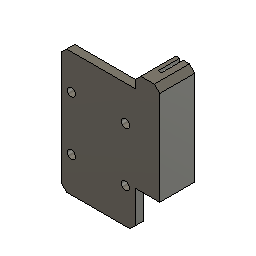
Placestation_Toolhead (Autodesk Fusion 360 archive; units mm, degrees)
design "Z-gantry-backplate-left-mgn12h"
part number: MGN12H-linear-rail-carriage
Autodesk Fusion 360 part; units mm, degrees
note: some values were not read from the file. Set by a fixed rule: which face or edge a step refers to.
sketch "Sketch4" plane through (0, 0, 122.6176) normal (0, 0, 1) x (1, 0, 0)
  line L0 (15.9, 225.325) -> (3.9, 225.325)
  line L1 (3.9, 225.325) -> (3.9, 192.925)
  line L2 (3.9, 192.925) -> (15.9, 192.925)
  line L3 (15.9, 192.925) -> (15.9, 225.325)
  line L4 (41.5656, 188.8314, 7.825) -> (5.0656, 188.8314, 7.825)
  line L5 (5.0656, 188.8314, 7.825) -> (5.0656, 234.6853, 9.8822)
  line L6 (5.0656, 234.6853, 9.8822) -> (41.5656, 234.6853, 9.8822)
  line L7 (41.5656, 234.6853, 9.8822) -> (41.5656, 188.8314, 7.825)
  line L8 (41.5656, 188.8314, 7.825) -> (5.0656, 234.6853, 9.8822) construction
  line L9 (5.0656, 188.8314, 7.825) -> (41.5656, 234.6853, 9.8822) construction
  line L10 (23.4, 192.925, -0.2) -> (23.4, 225.325, -0.2)
  circle A0 through (21.45, 219.125, 0.1295) (19.125, 220.4673, 0.1295) (19.125, 217.7827, 0.1295)
  circle A1 through (21.1295, 219.125, 0.1295) (19.2852, 220.1898, 0.1295) (19.2852, 218.0602, 0.1295)
  circle A2 through (1.45, 219.125, 0.1295) (-0.875, 220.4673, 0.1295) (-0.875, 217.7827, 0.1295)
  circle A3 through (1.1295, 219.125, 0.1295) (-0.7147, 220.1898, 0.1295) (-0.7147, 218.0602, 0.1295)
  circle A4 through (21.45, 199.125, 0.1295) (19.125, 200.4673, 0.1295) (19.125, 197.7827, 0.1295)
  circle A5 through (21.1295, 199.125, 0.1295) (19.2852, 200.1898, 0.1295) (19.2852, 198.0602, 0.1295)
  circle A6 through (1.45, 199.125, 0.1295) (-0.875, 200.4673, 0.1295) (-0.875, 197.7827, 0.1295)
  circle A7 through (1.1295, 199.125, 0.1295) (-0.7147, 200.1898, 0.1295) (-0.7147, 198.0602, 0.1295)
  point P0 (23.3156, 211.7584)
  point P1 (23.3156, 211.7584)
  dimension "d15" = 16.2
  dimension "d17" = 36.5
  dimension "d18" = 45.9
  dimension "d19" = 9.054
  dimension "d21" = 3.1
  dimension "d22" = 3.1
  dimension "d23" = 3.1
  dimension "d24" = 3.1
  constraint coincident P1 P0
  measures "d15" distance of L0 P1
sketch "Sketch5" plane through (10.1103, 0, 115.5608) normal (-0.087156, 0, -0.996195) x (-0.996195, 0, 0.087156)
  line L0 (5.3253, 232.125) -> (4.9573, 232.125)
  line L1 (4.9573, 232.125) -> (4.9573, 186.125)
  line L2 (4.9573, 186.125) -> (5.3253, 186.125)
  line L3 (5.3253, 186.125) -> (5.3253, 232.125)
sketch "Sketch6" plane through (0, 0, 123.0176) normal (0, 0, 1) x (1, 0, 0)
  line L0 (22.8, 225.325) -> (16.3, 225.325)
  line L1 (16.3, 225.325) -> (16.3, 192.925)
  line L2 (16.3, 192.925) -> (22.8, 192.925)
  line L3 (22.8, 192.925) -> (22.8, 225.325)
  circle A0 centre (19.9, 219.125) radius 1.5
  circle A1 centre (19.9, 199.125) radius 1.5
sketch "Sketch7" plane through (0, 0, 123.0176) normal (0, 0, 1) x (1, 0, 0)
  line L0 (3.5, 225.325) -> (-3, 225.325)
  line L1 (-3, 225.325) -> (-3, 192.925)
  line L2 (-3, 192.925) -> (3.5, 192.925)
  line L3 (3.5, 192.925) -> (3.5, 225.325)
  circle A0 centre (-0.1, 219.125) radius 1.5
  circle A1 centre (-0.1, 199.125) radius 1.5
sketch "Sketch8" plane through (0, -5.461, 121.726) normal (0, 0.044818, -0.998995) x (-1, 0, 0)
  line L0 (-5.0656, 240.3879) -> (-41.5656, 240.3879)
  line L1 (-41.5656, 240.3879) -> (-41.5656, 194.4879)
  line L2 (-41.5656, 194.4879) -> (-5.0656, 194.4879)
  line L3 (-5.0656, 194.4879) -> (-5.0656, 240.3879)
  line L4 (-41.5656, 235.3879) -> (-33.6656, 235.3879)
  line L5 (-33.6656, 235.3879) -> (-33.6656, 194.4879)
  line L6 (-33.6656, 194.4879) -> (-41.5656, 194.4879)
  line L7 (-41.5656, 194.4879) -> (-41.5656, 235.3879)
  line L8 (-39.5659, 194.4879) -> (-41.5656, 196.4876)
  line L9 (-39.5659, 194.4879) -> (-32.9811, 194.4879) construction
  line L10 (-35.6653, 194.4879) -> (-33.6656, 196.4876)
  line L11 (-35.6653, 194.4879) -> (-22.4855, 194.4879) construction
  line L12 (-39.5659, 240.3879) -> (-41.5656, 238.3882)
  line L13 (-39.5659, 240.3879) -> (-32.2699, 240.3879) construction
  dimension "d33" = 7.9
  dimension "d34" = 40.9
  dimension "d36" = 5
  dimension "d37" = 45
  dimension "d38" = 2.828
  dimension "d39" = 45
  dimension "d40" = 2.828
  dimension "d41" = 45
  dimension "d42" = 2.828
  constraint horizontal L4
  constraint vertical L5
  constraint horizontal L6
  constraint vertical L7
  constraint coincident L1 L4.start
  constraint horizontal L9
  constraint coincident L2 L8.start
  constraint coincident L1 L8.end
  constraint horizontal L11
  constraint coincident L2 L10.start
  constraint coincident L5 L10.end
  constraint horizontal L13
  constraint coincident L0 L12.start
  constraint coincident L1 L12.end
  measures "d33" distance of L4.start L4.end
  measures "d34" distance of L4.start L1.end
  measures "d36" distance of L0 L4
  measures "d37" angle of L8 L9
  measures "d38" distance of L8.start L8.end
  measures "d39" angle of L10 L11
  measures "d40" distance of L10.start L10.end
  measures "d41" angle of L12 L13
  measures "d42" distance of L12.start L12.end
sketch "Sketch9" plane through (0, 235.1513, 10.5496) normal (0, 0.998995, 0.044818) x (-1, 0, 0)
  line L0 (-41.5656, 121.8485) -> (-41.5656, 111.8485)
  line L1 (-41.5656, 111.8485) -> (-33.6656, 111.8485)
  line L2 (-33.6656, 111.8485) -> (-33.6656, 121.8485)
  circle A0 centre (-27.5974, 117.8274) radius 1.575
  circle A1 centre (-27.5974, 117.8274) radius 1.25
  line L3 (-33.6656, 121.8485) -> (-41.5656, 121.8485)
  dimension "d52" = 3.15
  dimension "d53" = 2.5
  constraint concentric A0 A1
  measures "d52" diameter of A0
  measures "d53" diameter of A1
sketch "Sketch10" plane through (0, -5.461, 121.726) normal (0, 0.044818, -0.998995) x (-1, 0, 0)
  line L0 (-39.5659, 240.3879) -> (-41.5656, 238.3882)
  line L1 (-41.5656, 238.3882) -> (-41.5656, 235.3879)
  line L2 (-41.5656, 235.3879) -> (-33.6656, 235.3879)
  line L3 (-33.6656, 235.3879) -> (-33.6656, 196.4876)
  line L4 (-33.6656, 196.4876) -> (-35.6653, 194.4879)
  line L5 (-35.6653, 194.4879) -> (-5.0656, 194.4879)
  line L6 (-5.0656, 194.4879) -> (-5.0656, 240.3879)
  line L7 (-5.0656, 240.3879) -> (-39.5659, 240.3879)
  line L8 (-7.0653, 194.4879) -> (-5.0656, 196.4876)
  line L9 (-7.0653, 194.4879) -> (-6.662, 194.4879) construction
  dimension "d57" = 45
  dimension "d58" = 2.828
  constraint horizontal L9
  constraint coincident L5 L8.start
  constraint coincident L6 L8.end
  measures "d57" angle of L8 L9
  measures "d58" distance of L8.start L8.end
sketch "Sketch11" plane through (0, -5.461, 121.726) normal (0, 0.044818, -0.998995) x (-1, 0, 0)
  line L0 (-39.5659, 240.3879) -> (-41.5656, 238.3882)
  line L1 (-41.5656, 238.3882) -> (-41.5656, 235.3879)
  line L2 (-41.5656, 235.3879) -> (-33.6656, 235.3879)
  line L3 (-33.6656, 235.3879) -> (-33.6656, 196.4876)
  line L4 (-33.6656, 196.4876) -> (-35.6653, 194.4879)
  line L5 (-35.6653, 194.4879) -> (-5.0656, 194.4879)
  line L6 (-5.0656, 194.4879) -> (-5.0656, 240.3879)
  line L7 (-5.0656, 240.3879) -> (-39.5659, 240.3879)
  line L8 (-5.0656, 204.4879) -> (-14.0656, 204.4879)
  line L9 (-14.0656, 204.4879) -> (-14.0656, 245.3879)
  line L10 (-14.0656, 245.3879) -> (-5.0656, 245.3879)
  line L11 (-5.0656, 245.3879) -> (-5.0656, 204.4879)
  line L12 (-7.0653, 204.4879) -> (-5.0656, 206.4876)
  line L13 (-7.0653, 204.4879) -> (12.9274, 204.4879) construction
  line L14 (-14.0656, 243.3882) -> (-12.0659, 245.3879)
  line L15 (-14.0656, 243.3882) -> (6.6806, 243.3882) construction
  line L16 (-5.0656, 243.3882) -> (-7.0653, 245.3879)
  line L17 (-5.0656, 243.3882) -> (10.0246, 243.3882) construction
  line L18 (-16.0653, 240.3879) -> (-14.0656, 242.3876)
  line L19 (-16.0653, 240.3879) -> (5.0782, 240.3879) construction
  dimension "d64" = 9
  dimension "d65" = 40.9
  dimension "d66" = 10
  dimension "d67" = 45
  dimension "d68" = 2.828
  dimension "d69" = 45
  dimension "d70" = 2.828
  dimension "d71" = 45
  dimension "d72" = 2.828
  dimension "d75" = 45
  dimension "d76" = 2.828
  constraint horizontal L8
  constraint vertical L9
  constraint horizontal L10
  constraint vertical L11
  constraint coincident L6 L8.start
  constraint horizontal L13
  constraint coincident L8 L12.start
  constraint coincident L6 L12.end
  constraint horizontal L15
  constraint coincident L9 L14.start
  constraint coincident L10 L14.end
  constraint horizontal L17
  constraint coincident L11 L16.start
  constraint coincident L10 L16.end
  constraint horizontal L19
  constraint coincident L7 L18.start
  constraint coincident L9 L18.end
  measures "d64" distance of L8.start L8.end
  measures "d65" distance of L8.start L10.end
  measures "d66" distance of L5 L8
  measures "d67" angle of L12 L13
  measures "d68" distance of L12.start L12.end
  measures "d69" angle of L14 L15
  measures "d70" distance of L14.start L14.end
  measures "d71" angle of L16 L17
  measures "d72" distance of L16.start L16.end
  measures "d75" angle of L18 L19
  measures "d76" distance of L18.start L18.end
sketch "Sketch12" plane through (0, -5.0128, 111.7361) normal (0, 0.044818, -0.998995) x (-1, 0, 0)
  line L0 (-5.0656, 206.4876) -> (-5.0656, 243.3882)
  line L1 (-5.0656, 243.3882) -> (-7.0653, 245.3879)
  line L2 (-7.0653, 245.3879) -> (-12.0659, 245.3879)
  line L3 (-12.0659, 245.3879) -> (-14.0656, 243.3882)
  line L4 (-14.0656, 243.3882) -> (-14.0656, 204.4879)
  line L5 (-14.0656, 204.4879) -> (-7.0653, 204.4879)
  line L6 (-7.0653, 204.4879) -> (-5.0656, 206.4876)
  line L7 (-10.6656, 245.3879) -> (-9.3656, 245.3879)
  line L8 (-9.3656, 245.3879) -> (-9.3656, 204.4879)
  line L9 (-9.3656, 204.4879) -> (-10.6656, 204.4879)
  line L10 (-10.6656, 204.4879) -> (-10.6656, 245.3879)
  dimension "d81" = 1.3
  dimension "d82" = 40.9
  dimension "d83" = 3.4
  constraint horizontal L7
  constraint vertical L8
  constraint horizontal L9
  constraint vertical L10
  constraint coincident L2 L7.start
  measures "d81" distance of L7.start L7.end
  measures "d82" distance of L7.start L9.end
  measures "d83" distance of L4 L10
sketch "Sketch13" plane through (0, -5.0128, 111.7361) normal (0, 0.044818, -0.998995) x (-1, 0, 0)
  line L0 (-9.3656, 245.3879) -> (-9.3656, 204.4879)
  line L1 (-9.3656, 204.4879) -> (-7.0653, 204.4879)
  line L2 (-7.0653, 204.4879) -> (-5.0656, 206.4876)
  line L3 (-5.0656, 206.4876) -> (-5.0656, 243.3882)
  line L4 (-5.0656, 243.3882) -> (-7.0653, 245.3879)
  line L5 (-7.0653, 245.3879) -> (-9.3656, 245.3879)
  arc A0 (-9.3656, 245.3879) -> (-9.3656, 244.3879) centre (-9.3656, 244.8879) ccw
  arc A1 (-9.3656, 245.3879) -> (-9.3656, 244.3879) centre (-9.349, 244.8879) ccw
  dimension "d86" = 1
  dimension "d87" = 1
  constraint tangent L5 A0
  constraint coincident L0.start L5.end
  constraint coincident L0 L5.end
  measures "d86" distance of L0.start A0.end
  measures "d87" distance of A0.end L0.start
pattern_linear "R-Pattern2" [no effect]
sketch "Sketch14" plane through (0, -5.461, 121.726) normal (0, 0.044818, -0.998995) x (-1, 0, 0)
  line L0 (-14.0656, 243.3882) -> (-14.0656, 242.3876)
  line L1 (-14.0656, 242.3876) -> (-16.0653, 240.3879)
  line L2 (-14.0656, 243.3882) -> (-14.0656, 194.4879)
  line L3 (-14.0656, 202.4882) -> (-12.0659, 204.4879)
  line L4 (-14.0656, 202.4882) -> (6.6806, 202.4882) construction
  line L5 (-16.0653, 194.4879) -> (-14.0656, 196.4876)
  line L6 (-16.0653, 194.4879) -> (4.3386, 194.4879) construction
  line L7 (-12.0659, 204.4879) -> (-7.0653, 204.4879)
  line L8 (-7.0653, 204.4879) -> (-5.0656, 206.4876)
  line L9 (-5.0656, 206.4876) -> (-5.0656, 194.4879)
  line L10 (-5.0656, 194.4879) -> (-14.0656, 194.4879)
  line L11 (-16.0653, 240.3879) -> (-5.0656, 240.3879)
  line L12 (-5.0656, 243.3882) -> (-7.0653, 245.3879)
  line L13 (-7.0653, 245.3879) -> (-12.0659, 245.3879)
  line L14 (-12.0659, 245.3879) -> (-14.0656, 243.3882)
  line L15 (-5.0656, 240.3879) -> (-5.0656, 243.3882)
  dimension "d101" = 45
  dimension "d102" = 2.828
  dimension "d103" = 45
  dimension "d104" = 2.828
  constraint coincident L0.start L2.start
  constraint horizontal L4
  constraint coincident L2 L3.start
  constraint horizontal L6
  constraint coincident L2 L5.end
  measures "d101" angle of L3 L4
  measures "d102" distance of L3.start L3.end
  measures "d103" angle of L5 L6
  measures "d104" distance of L5.start L5.end
sketch "1st for left Sketch" plane through (0, 0, 122.6176) normal (0, 0, 1) x (1, 0, 0)
  line L0 (15.9, 225.325) -> (3.9, 225.325)
  line L1 (3.9, 225.325) -> (3.9, 192.925)
  line L2 (3.9, 192.925) -> (15.9, 192.925)
  line L3 (15.9, 192.925) -> (15.9, 225.325)
  line L4 (23.4, 192.925, -0.2) -> (23.4, 225.325, -0.2)
  line L5 (32.5981, 232.075, -0.0049) -> (-3.9019, 232.075, -0.0049)
  line L6 (-3.9019, 232.075, -0.0049) -> (-3.9019, 186.175, -0.0005)
  line L7 (-3.9019, 186.175) -> (32.5981, 186.175)
  line L8 (32.5981, 186.175, -0.0005) -> (32.5981, 232.075, -0.0049)
  line L9 (32.5981, 232.075, -0.0049) -> (-3.9019, 186.175, -0.0005) construction
  line L10 (-3.9019, 232.075, -0.0049) -> (32.5981, 186.175, -0.0005) construction
  point P0 (14.3481, 209.125)
  point P1 (14.3481, 209.125)
  dimension "d109" = 16.2
  dimension "d110" = 9.054
  dimension "d111" = 36.5
  dimension "d112" = 45.9
  constraint coincident P1 P0
  measures "d109" distance of L0 P1
  measures "d111" distance of L7.start L7.end
sketch "1st for left Sketch (curves on the plane with normal 0, 0.0001, 1 at 0.0173 mm)" plane through (0, 0, 122.6349) normal (0, 0.000096, 1) x (-1, 0, 0)
  line L0 (-32.5981, -232.075) -> (3.9019, -232.075)
  line L1 (3.9019, -232.075) -> (3.9019, -186.175)
  line L2 (3.9019, -186.175) -> (-32.5981, -186.175)
  line L3 (-32.5981, -186.175) -> (-32.5981, -232.075)
  line L4 (-32.5981, -232.075) -> (3.9019, -186.175) construction
  line L5 (3.9019, -232.075) -> (-32.5981, -186.175) construction
extrude "Extrude16" add sketch "1st for left Sketch (curves on the plane with normal 0, 0.0001, 1 at 0.0173 mm)" along normal blind 3
sketch "Sketch16" plane through (0, 0, 123.0176) normal (0, 0, 1) x (1, 0, 0)
  line L0 (3.5, 225.325) -> (-3, 225.325)
  line L1 (-3, 225.325) -> (-3, 192.925)
  line L2 (-3, 192.925) -> (3.5, 192.925)
  line L3 (3.5, 192.925) -> (3.5, 225.325)
  circle A0 centre (-0.1, 219.125) radius 1.5
  circle A1 centre (-0.1, 199.125) radius 1.5
sketch "Sketch17" plane through (0, 0, 123.0176) normal (0, 0, 1) x (1, 0, 0)
  line L0 (22.8, 225.325) -> (16.3, 225.325)
  line L1 (16.3, 225.325) -> (16.3, 192.925)
  line L2 (16.3, 192.925) -> (22.8, 192.925)
  line L3 (22.8, 192.925) -> (22.8, 225.325)
  circle A0 centre (19.9, 219.125) radius 1.5
  circle A1 centre (19.9, 199.125) radius 1.5
extrude "Extrude17" cut sketch "Sketch16" sketch "Sketch17" along normal blind 3 contours A0 | A1 of sketch 2 contours A0 | A1
extrude "Extrude18" cut 4 faces at (-0.5131, 218.6943, 123.0176) (-0.5131, 198.6943, 123.0176) (19.4869, 218.6943, 123.0176) (19.4869, 198.6943, 123.0176) along direction (0, 0, -1) blind 1
sketch "Sketch18" plane through (0, 0.0118, 122.6349) normal (0, -0.000096, -1) x (-1, 0, 0)
  ellipse E0 centre (-19.9, 199.1132) end of major axis (-19.9, 197.6132) minor radius 1.5
  ellipse E1 centre (0.1, 219.1132) end of major axis (0.1, 217.6132) minor radius 1.5
  ellipse E2 centre (-19.9, 219.1132) end of major axis (-19.9, 217.6132) minor radius 1.5
  ellipse E3 centre (0.1, 199.1132) end of major axis (0.1, 197.6132) minor radius 1.5
  line L0 (-32.5981, 232.0632) -> (-32.5981, 186.1632)
  line L1 (-32.5981, 186.1632) -> (3.9019, 186.1632)
  line L2 (3.9019, 186.1632) -> (3.9019, 232.0632)
  line L3 (3.9019, 232.0632) -> (-32.5981, 232.0632)
  line L4 (1.9022, 186.1632) -> (3.9019, 188.1629)
  line L5 (1.9022, 186.1632) -> (3.9019, 186.1632) construction
  line L6 (1.9022, 232.0632) -> (3.9019, 230.0635)
  line L7 (1.9022, 232.0632) -> (5.2821, 232.0632) construction
  line L8 (-30.5985, 186.1632) -> (-32.5981, 188.1629)
  line L9 (-30.5985, 186.1632) -> (-32.7199, 186.1632) construction
  dimension "d119" = 45
  dimension "d120" = 2.828
  dimension "d121" = 45
  dimension "d122" = 2.828
  dimension "d123" = 45
  dimension "d124" = 2.828
  constraint horizontal L5
  constraint coincident L1 L4.start
  constraint coincident L2 L4.end
  constraint horizontal L7
  constraint coincident L3 L6.start
  constraint coincident L2 L6.end
  constraint horizontal L9
  constraint coincident L1 L8.start
  constraint coincident L0 L8.end
  measures "d119" angle of L4 L5
  measures "d120" distance of L4.start L4.end
  measures "d121" angle of L6 L7
  measures "d122" distance of L6.start L6.end
  measures "d123" angle of L8 L9
  measures "d124" distance of L8.start L8.end
extrude "Extrude19" cut sketch "Sketch18" against normal blind 3 contours L0 L1 L8 | L2 L3 L6 | L1 L2 L4
sketch "Sketch19" plane through (0, 0.0118, 122.6349) normal (0, -0.000096, -1) x (-1, 0, 0)
  ellipse E0 centre (0.1, 199.1132) end of major axis (0.1, 197.6132) minor radius 1.5
  ellipse E1 centre (-19.9, 219.1132) end of major axis (-19.9, 217.6132) minor radius 1.5
  ellipse E2 centre (0.1, 219.1132) end of major axis (0.1, 217.6132) minor radius 1.5
  ellipse E3 centre (-19.9, 199.1132) end of major axis (-19.9, 197.6132) minor radius 1.5
  line L0 (-32.5981, 188.1629) -> (-30.5985, 186.1632)
  line L1 (-30.5985, 186.1632) -> (1.9022, 186.1632)
  line L2 (1.9022, 186.1632) -> (3.9019, 188.1629)
  line L3 (3.9019, 188.1629) -> (3.9019, 230.0635)
  line L4 (3.9019, 230.0635) -> (1.9022, 232.0632)
  line L5 (1.9022, 232.0632) -> (-32.5981, 232.0632)
  line L6 (-32.5981, 232.0632) -> (-32.5981, 188.1629)
  line L7 (-32.5981, 237.0632) -> (-23.5981, 237.0632)
  line L8 (-23.5981, 237.0632) -> (-23.5981, 196.1632)
  line L9 (-23.5981, 196.1632) -> (-32.5981, 196.1632)
  line L10 (-32.5981, 196.1632) -> (-32.5981, 237.0632)
  line L11 (-30.5985, 196.1632) -> (-32.5981, 198.1629)
  line L12 (-30.5985, 196.1632) -> (-33.0345, 196.1632) construction
  line L13 (-32.5981, 235.0635) -> (-30.5985, 237.0632)
  line L14 (-32.5981, 235.0635) -> (-29.7701, 235.0635) construction
  line L15 (-23.5981, 235.0635) -> (-25.5978, 237.0632)
  line L16 (-23.5981, 235.0635) -> (-26.4261, 235.0635) construction
  dimension "d127" = 9
  dimension "d128" = 40.9
  dimension "d129" = 10
  dimension "d130" = 45
  dimension "d131" = 2.828
  dimension "d132" = 45
  dimension "d133" = 2.828
  dimension "d134" = 45
  dimension "d135" = 2.828
  constraint horizontal L7
  constraint vertical L8
  constraint horizontal L9
  constraint vertical L10
  constraint coincident L6 L7.start
  constraint horizontal L12
  constraint coincident L9 L11.start
  constraint coincident L6 L11.end
  constraint horizontal L14
  constraint coincident L10 L13.start
  constraint coincident L7 L13.end
  constraint horizontal L16
  constraint coincident L8 L15.start
  constraint coincident L7 L15.end
  measures "d127" distance of L7.start L7.end
  measures "d128" distance of L7.start L9.end
  measures "d129" distance of L1 L9
  measures "d130" angle of L11 L12
  measures "d131" distance of L11.start L11.end
  measures "d132" angle of L13 L14
  measures "d133" distance of L13.start L13.end
  measures "d134" angle of L15 L16
  measures "d135" distance of L15.start L15.end
extrude "Extrude20" add sketch "Sketch19" along normal blind 10 contours L5 L6 L8 L9 L10 L11 | L5 L7 L8 L10 L13 L15
sketch "Sketch20" plane through (0, 0.0108, 112.6349) normal (0, -0.000096, -1) x (-1, 0, 0)
  line L0 (-23.5981, 196.1632) -> (-23.5981, 235.0635)
  line L1 (-23.5981, 235.0635) -> (-25.5978, 237.0632)
  line L2 (-25.5978, 237.0632) -> (-30.5985, 237.0632)
  line L3 (-30.5985, 237.0632) -> (-32.5981, 235.0635)
  line L4 (-32.5981, 235.0635) -> (-32.5981, 198.1629)
  line L5 (-32.5981, 198.1629) -> (-30.5985, 196.1632)
  line L6 (-30.5985, 196.1632) -> (-23.5981, 196.1632)
  line L7 (-28.2981, 237.0632) -> (-26.9981, 237.0632)
  line L8 (-26.9981, 237.0632) -> (-26.9981, 196.1632)
  line L9 (-26.9981, 196.1632) -> (-28.2981, 196.1632)
  line L10 (-28.2981, 196.1632) -> (-28.2981, 237.0632)
  arc A0 (-28.2981, 236.0632) -> (-28.2981, 237.0632) centre (-28.3185, 236.5632) ccw
  arc A1 (-28.2981, 236.0632) -> (-28.2981, 235.0632) centre (-28.2778, 235.5632) ccw
  dimension "d138" = 1.3
  dimension "d139" = 40.9
  dimension "d140" = 3.4
  dimension "d141" = 1
  dimension "d142" = 1
  constraint horizontal L7
  constraint vertical L8
  constraint horizontal L9
  constraint vertical L10
  constraint coincident L2 L7.start
  constraint tangent A0 A1
  measures "d138" distance of L7.start L7.end
  measures "d139" distance of L7.start L9.end
  measures "d140" distance of L0 L8
  measures "d141" distance of L7.start A0.start
  measures "d142" distance of A0.start A1.end
extrude "Extrude21" add 1 faces at (28.9316, 233.7417, 122.6125) along direction (0, 0.000096, 1) blind 3
extrude "Extrude22" cut sketch "Sketch20" against normal blind 10 contours L2 L6 L7 L8 L9 L10 A0 | L10 A0
extrude "Extrude23" add sketch "Sketch20" against normal blind 10 contours L10 A0
extrude "Extrude24" cut sketch "Sketch20" against normal blind 10 contours L10 A1
pattern_linear "R-Pattern3" count 21 spacing 2 along (0, -1, 0.000096) of "Extrude23"
pattern_linear "R-Pattern4" count 21 spacing 2 along (0, -1, 0.000096) of "Extrude24"
extrude "Extrude25" cut 1 faces at (28.2981, 196.1077, 115.9494) along direction (-1, 0, 0) blind 0.9
sketch "Sketch21" plane through (0, 0.0118, 122.6349) normal (0, -0.000096, -1) x (-1, 0, 0)
  line L0 (-28.0178, 196.1632) -> (-30.5985, 196.1632)
  line L1 (-30.5985, 196.1632) -> (-32.5981, 198.1629)
  line L2 (-32.5981, 198.1629) -> (-32.5981, 188.1629)
  line L3 (-32.5981, 188.1629) -> (-30.5985, 186.1632)
  line L4 (-30.5985, 186.1632) -> (1.9022, 186.1632)
  line L5 (1.9022, 186.1632) -> (3.9019, 188.1629)
  line L6 (3.9019, 188.1629) -> (3.9019, 230.0635)
  line L7 (3.9019, 230.0635) -> (1.9022, 232.0632)
  line L8 (1.9022, 232.0632) -> (-23.5981, 232.0632)
  line L9 (-23.5981, 232.0632) -> (-23.5981, 196.1632)
  line L10 (-23.5981, 196.1632) -> (-26.9981, 196.1632)
  line L11 (-26.9981, 196.1632) -> (-26.9981, 237.0632)
  line L12 (-26.9981, 237.0632) -> (-28.2981, 237.0632)
  arc A0 (-28.2981, 236.0632) -> (-28.2981, 237.0632) centre (-28.3185, 236.5632) ccw
  arc A1 (-28.2981, 236.0632) -> (-28.2981, 235.0632) centre (-28.2778, 235.5632) ccw
  arc A2 (-28.2981, 234.0632) -> (-28.2981, 235.0632) centre (-28.3185, 234.5632) ccw
  arc A3 (-28.2981, 234.0632) -> (-28.2981, 233.0632) centre (-28.2778, 233.5632) ccw
  arc A4 (-28.2981, 232.0632) -> (-28.2981, 233.0632) centre (-28.3185, 232.5632) ccw
  arc A5 (-28.2981, 232.0632) -> (-28.2981, 231.0632) centre (-28.2778, 231.5632) ccw
  arc A6 (-28.2981, 230.0632) -> (-28.2981, 231.0632) centre (-28.3185, 230.5632) ccw
  arc A7 (-28.2981, 230.0632) -> (-28.2981, 229.0632) centre (-28.2778, 229.5632) ccw
  arc A8 (-28.2981, 228.0632) -> (-28.2981, 229.0632) centre (-28.3185, 228.5632) ccw
  arc A9 (-28.2981, 228.0632) -> (-28.2981, 227.0632) centre (-28.2778, 227.5632) ccw
  arc A10 (-28.2981, 226.0632) -> (-28.2981, 227.0632) centre (-28.3185, 226.5632) ccw
  arc A11 (-28.2981, 226.0632) -> (-28.2981, 225.0632) centre (-28.2778, 225.5632) ccw
  arc A12 (-28.2981, 224.0632) -> (-28.2981, 225.0632) centre (-28.3185, 224.5632) ccw
  arc A13 (-28.2981, 224.0632) -> (-28.2981, 223.0632) centre (-28.2778, 223.5632) ccw
  arc A14 (-28.2981, 222.0632) -> (-28.2981, 223.0632) centre (-28.3185, 222.5632) ccw
  arc A15 (-28.2981, 222.0632) -> (-28.2981, 221.0632) centre (-28.2778, 221.5632) ccw
  arc A16 (-28.2981, 220.0632) -> (-28.2981, 221.0632) centre (-28.3185, 220.5632) ccw
  arc A17 (-28.2981, 220.0632) -> (-28.2981, 219.0632) centre (-28.2778, 219.5632) ccw
  arc A18 (-28.2981, 218.0632) -> (-28.2981, 219.0632) centre (-28.3185, 218.5632) ccw
  arc A19 (-28.2981, 218.0632) -> (-28.2981, 217.0632) centre (-28.2778, 217.5632) ccw
  arc A20 (-28.2981, 216.0632) -> (-28.2981, 217.0632) centre (-28.3185, 216.5632) ccw
  arc A21 (-28.2981, 216.0632) -> (-28.2981, 215.0632) centre (-28.2778, 215.5632) ccw
  arc A22 (-28.2981, 214.0632) -> (-28.2981, 215.0632) centre (-28.3185, 214.5632) ccw
  arc A23 (-28.2981, 214.0632) -> (-28.2981, 213.0632) centre (-28.2778, 213.5632) ccw
  arc A24 (-28.2981, 212.0632) -> (-28.2981, 213.0632) centre (-28.3185, 212.5632) ccw
  arc A25 (-28.2981, 212.0632) -> (-28.2981, 211.0632) centre (-28.2778, 211.5632) ccw
  arc A26 (-28.2981, 210.0632) -> (-28.2981, 211.0632) centre (-28.3185, 210.5632) ccw
  arc A27 (-28.2981, 210.0632) -> (-28.2981, 209.0632) centre (-28.2778, 209.5632) ccw
  arc A28 (-28.2981, 208.0632) -> (-28.2981, 209.0632) centre (-28.3185, 208.5632) ccw
  arc A29 (-28.2981, 208.0632) -> (-28.2981, 207.0632) centre (-28.2778, 207.5632) ccw
  arc A30 (-28.2981, 206.0632) -> (-28.2981, 207.0632) centre (-28.3185, 206.5632) ccw
  arc A31 (-28.2981, 206.0632) -> (-28.2981, 205.0632) centre (-28.2778, 205.5632) ccw
  arc A32 (-28.2981, 204.0632) -> (-28.2981, 205.0632) centre (-28.3185, 204.5632) ccw
  arc A33 (-28.2981, 204.0632) -> (-28.2981, 203.0632) centre (-28.2778, 203.5632) ccw
  arc A34 (-28.2981, 202.0632) -> (-28.2981, 203.0632) centre (-28.3185, 202.5632) ccw
  arc A35 (-28.2981, 202.0632) -> (-28.2981, 201.0632) centre (-28.2778, 201.5632) ccw
  arc A36 (-28.2981, 200.0632) -> (-28.2981, 201.0632) centre (-28.3185, 200.5632) ccw
  arc A37 (-28.2981, 200.0632) -> (-28.2981, 199.0632) centre (-28.2778, 199.5632) ccw
  arc A38 (-28.2981, 198.0632) -> (-28.2981, 199.0632) centre (-28.3185, 198.5632) ccw
  arc A39 (-28.2981, 198.0632) -> (-28.2981, 197.0632) centre (-28.2778, 197.5632) ccw
  arc A40 (-28.0178, 196.1632) -> (-28.2981, 197.0632) centre (-28.3185, 196.5632) ccw
  ellipse E0 centre (0.1, 199.1132) end of major axis (0.1, 197.6132) minor radius 1.5
  ellipse E1 centre (-19.9, 219.1132) end of major axis (-19.9, 217.6132) minor radius 1.5
  ellipse E2 centre (0.1, 219.1132) end of major axis (0.1, 217.6132) minor radius 1.5
  ellipse E3 centre (-19.9, 199.1132) end of major axis (-19.9, 197.6132) minor radius 1.5
  line L13 (-23.5981, 196.1632) -> (-23.5981, 186.1632)
  line L14 (-23.5981, 196.1632) -> (-30.5985, 196.1632)
  line L15 (-30.5985, 196.1632) -> (-32.5981, 198.1629)
  line L16 (-32.5981, 198.1629) -> (-32.5981, 188.1629)
  line L17 (-32.5981, 188.1629) -> (-30.5985, 186.1632)
  line L18 (-30.5985, 186.1632) -> (-23.5981, 186.1632)
  line L19 (-23.5981, 188.1629) -> (-21.5985, 186.1632)
  line L20 (-23.5981, 188.1629) -> (-20.7701, 188.1629) construction
  dimension "d161" = 45
  dimension "d162" = 2.828
  constraint coincident L9.end L10.start
  constraint coincident L4 L13.end
  constraint perpendicular L4 L13
  constraint coincident L0.end L1.start
  constraint coincident L1.end L2.start
  constraint coincident L2.end L3.start
  constraint coincident L3.end L4.start
  constraint horizontal L20
  constraint coincident L13 L19.start
  constraint coincident L4 L19.end
  measures "d161" angle of L19 L20
  measures "d162" distance of L19.start L19.end
extrude "Extrude26" cut sketch "Sketch21" against normal blind 3 contours L0 L1 L2 L3 L4 L10 L13 L14 L15 L16 L17 L18 | L4 L13 L19
sketch "Sketch22" plane through (0, 0.0121, 125.6349) normal (0, 0.000096, 1) x (1, 0, 0)
  line L0 (21.5985, 186.1632) -> (23.5981, 188.1629)
  line L1 (23.5981, 188.1629) -> (23.5981, 196.1632)
  line L2 (23.5981, 196.1632) -> (30.5985, 196.1632)
  line L3 (30.5985, 196.1632) -> (32.5981, 198.1629)
  line L4 (32.5981, 198.1629) -> (32.5981, 235.0635)
  line L5 (32.5981, 235.0635) -> (30.5985, 237.0632)
  line L6 (30.5985, 237.0632) -> (25.5978, 237.0632)
  line L7 (25.5978, 237.0632) -> (23.5981, 235.0635)
  line L8 (23.5981, 235.0635) -> (23.5981, 232.0632)
  line L9 (23.5981, 232.0632) -> (-1.9022, 232.0632)
  line L10 (-1.9022, 232.0632) -> (-3.9019, 230.0635)
  line L11 (-3.9019, 230.0635) -> (-3.9019, 188.1629)
  line L12 (-3.9019, 188.1629) -> (-1.9022, 186.1632)
  line L13 (-1.9022, 186.1632) -> (21.5985, 186.1632)
  ellipse E0 centre (19.9, 219.1129) end of major axis (19.9, 220.6129) minor radius 1.5
  ellipse E1 centre (-0.1, 219.1129) end of major axis (-0.1, 220.6129) minor radius 1.5
  ellipse E2 centre (-0.1, 199.1129) end of major axis (-0.1, 200.6129) minor radius 1.5
  ellipse E3 centre (19.9, 199.1129) end of major axis (19.9, 200.6129) minor radius 1.5
  line L14 (23.5981, 196.1632) -> (23.5981, 200.1632)
  line L15 (23.5981, 200.1632) -> (32.5981, 200.1632)
  dimension "d165" = 4
  constraint coincident L1.end L2.start
  constraint perpendicular L2 L14
  constraint coincident L4 L15.end
  constraint perpendicular L4 L15
  measures "d165" distance of L1.end L14.end
extrude "Extrude27" cut sketch "Sketch22" against normal blind 23 contours L2 L3 L4 L14 L15
extrude "Extrude28" add 1 faces at (27.2719, 215.2629, 122.6142) along direction (0, -0.000096, -1) blind 6
extrude "Extrude29" add 2 faces at (31.3244, 218.2863, 112.6139) (25.8648, 224.1075, 112.6134) along direction (0, -0.000096, -1) blind 3
extrude "Extrude30" cut 1 faces at (27.2719, 215.2623, 116.6142) along direction (0, 0.000096, 1) blind 4
extrude "Extrude31" cut 2 faces at (31.3244, 218.286, 109.6139) (25.8648, 224.1072, 109.6134) along direction (0, 0.000096, 1) blind 3
equation "L1 = 45.9 mm" comment "Length of Main Block"
equation "B1 = 27.5 mm + 9 mm" comment "Breadth of main block"
equation "SD1 = ( 32.4 / 2 ) * 1 mm" comment "Distance of center point frm top"
equation "SD2 = 14.054 mm - 5 mm" comment "distance of the center point from side"
equation "R1 = 3.1 mm" comment "Block holes"
equation "d15 = SD1"
equation "d17 = B1"
equation "d18 = L1"
equation "d19 = SD2"
equation "E1 = 3 mm"
equation "d21 = R1"
equation "d22 = R1"
equation "d23 = R1"
equation "d24 = R1"
equation "B2 = 7.9 mm" comment "Right side wing wwith screw breadth"
equation "L2 = L1 - 5 mm" comment "Lenght of right wing"
equation "d33 = B2"
equation "d34 = L2"
equation "SD3 = 5 mm" comment "Distance of right wing rectangle from top"
equation "d36 = SD3"
equation "E2 = 10 mm" comment "Right wing extrude"
equation "R2 = 2.5 mm" comment "right wing inner hole"
equation "R3 = 3.15 mm" comment "Right wing outer home"
equation "d52 = R3"
equation "d53 = R2"
equation "L3 = 40.9 mm" comment "Right wing length"
equation "B3 = 9 mm" comment "Right wing breadth"
equation "SD4 = 10 mm" comment "Distance of left wing from bottom"
equation "d64 = B3"
equation "d65 = L3"
equation "d66 = SD4"
equation "B4 = 1.3 mm" comment "Rectangle for gt2 belt teeth"
equation "SD5 = 3.4 mm" comment "distance of gt2 belt rectangle from inner side"
equation "d81 = B4"
equation "d82 = L2"
equation "d83 = SD5"
equation "d109 = SD1"
equation "d110 = SD2"
equation "d111 = B1"
equation "d112 = L1"
equation "d113 = E1"
equation "d127 = B3"
equation "d128 = L3"
equation "d129 = SD4"
equation "d136 = E2"
equation "d138 = B4"
equation "d139 = L3"
equation "d140 = SD5"
equation "d145 = -E2"
equation "d147 = -E2"
equation "d149 = -E2"
named bodies: "LeftBackplate"
